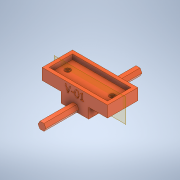
# Autodesk Inventor part: connectorToTubeBracketWithOffsetHexShaft-V01
Saved by Autodesk Inventor 2021.2 (Build 252289000, 289)
## iProperties
Created: 2020-07-23
Part Number: connectorToTubeBracketWithOffsetHexShaft-V01
Material: PBT Plastic
Document SubType Name: Modeling
Designer: robst
Density: 1.31 g/cm^3
Appearance: Smooth - Light Orange
Mass: 251.144 g
Surface Area: 396.963 cm^2
Volume: 251.144 cm^3
Author: robst
Autodesk Inventor part; units mm, degrees
ref_plane "YZ Plane" through (0, 0, 0) normal (1, 0, 0) x (0, 1, 0)
ref_plane "XZ Plane" through (0, 0, 0) normal (0, 1, 0) x (-1, 0, 0)
sketch "Sketch1" plane through (0, 0, 0) normal (0, 1, 0) x (-1, 0, 0)
  line L0 (53.975, 21.59) -> (-53.975, 21.59)
  line L1 (-53.975, 21.59) -> (-53.975, -21.59)
  line L2 (-53.975, -21.59) -> (53.975, -21.59)
  line L3 (53.975, -21.59) -> (53.975, 21.59)
  line L4 (53.975, 21.59) -> (-53.975, -21.59) construction
  line L5 (-53.975, 21.59) -> (53.975, -21.59) construction
  line L6 (60.325, 27.94) -> (-60.325, 27.94)
  line L7 (-60.325, 27.94) -> (-60.325, -27.94)
  line L8 (-60.325, -27.94) -> (60.325, -27.94)
  line L9 (60.325, -27.94) -> (60.325, 27.94)
  line L10 (60.325, 27.94) -> (-60.325, -27.94) construction
  line L11 (-60.325, 27.94) -> (60.325, -27.94) construction
  point P0 (0, 0)
  dimension "d0" = 43.18
  dimension "d1" = 107.95
  dimension "d2" = 6.35
  dimension "d3" = 6.35
  constraints: 24 end point, 4 midpoint, 4 parallel, 2 horizontal, 2 perpendicular
  measures "d0" distance of L0.end L1.end
  measures "d1" distance between parallel lines of L1 L3
  measures "d2" distance between parallel lines of L8 L2
  measures "d3" distance between parallel lines of L9 L3
extrude "Extrusion1" add sketch "Sketch1" against normal blind 12.065 contours L3 L2 L1 L0 | L9 L8 L7 L6
extrude "Extrusion2" add sketch "Sketch1" along normal blind 8.89
sketch "Sketch2" plane through (0, 0, 0) normal (0, 1, 0) x (1, 0, 0)
  line L0 (-53.975, 21.59) -> (-53.975, -21.59) construction
  line L1 (-53.975, 0) -> (53.975, 0) construction
  line L2 (53.975, -21.59) -> (53.975, 21.59) construction
  point P0 (0, 0)
  point P1 (-41.275, 0)
  point P2 (41.275, 0)
  dimension "d8" = 12.7
  dimension "d9" = 12.7
  constraints: 2 end point, 2 midpoint, 2 point on line
  measures "d8" distance from line of point (-41.275, 0) L0
  measures "d9" distance from line of point (41.275, 0) L2
hole "Hole1" at (-41.275, 0, 0) at (41.275, 0, 0) direction (0, -1, 0) diameter 5.1054 end through all counterbore diameter 10.16 counterbore depth 2.54 clearance for "Hex Machine Screw" size "#10" standard "Ansi Unified Screw Threads"
sketch "Sketch5" plane through (0, -12.065, 0) normal (0, -1, 0) x (1, 0, 0)
  line L0 (-25.4, -27.94) -> (25.4, -27.94)
  line L1 (25.4, -27.94) -> (25.4, 27.94)
  line L2 (25.4, 27.94) -> (-25.4, 27.94)
  line L3 (-25.4, 27.94) -> (-25.4, -27.94)
  line L4 (-25.4, -27.94) -> (25.4, 27.94) construction
  line L5 (25.4, -27.94) -> (-25.4, 27.94) construction
  point P0 (0, 0)
  dimension "d27" = 50.8
  dimension "d28" = 55.88
  constraints: 12 end point, 2 midpoint, 2 parallel, 1 horizontal, 1 perpendicular
  measures "d27" distance between parallel lines of L1 L3
  measures "d28" distance between parallel lines of L0 L2
extrude "Extrusion6" add sketch "Sketch5" along normal blind 19.05
sketch "Sketch11" plane through (-60.325, 8.89, 27.94) normal (0, 0, 1) x (1, 0, 0)
  line L0 (0, -20.955) -> (0, 0) construction
  line L1 (0, -10.4775) -> (120.65, -10.4775) construction
  line L2 (120.65, 0) -> (120.65, -20.955) construction
  line L3 (52.9098, -4.1275) -> (48.5358, -16.8275)
  line L4 (48.5358, -16.8275) -> (46.7142, -16.8275)
  line L5 (46.7142, -16.8275) -> (42.3402, -4.1275)
  line L6 (42.3402, -4.1275) -> (44.1515, -4.1275)
  line L7 (44.1515, -4.1275) -> (47.6713, -14.6765)
  line L8 (47.6713, -14.6765) -> (51.1911, -4.1275)
  line L9 (51.1911, -4.1275) -> (52.9098, -4.1275)
  line L10 (58.56, -12.0418) -> (53.7537, -12.0418)
  line L11 (53.7537, -12.0418) -> (53.7537, -10.4981)
  line L12 (53.7537, -10.4981) -> (58.56, -10.4981)
  line L13 (58.56, -10.4981) -> (58.56, -12.0418)
  spline S0 degree 2 poles (68.1519, -10.4775) (68.1519, -13.8944) (66.1656, -17.0951) (64.0969, -17.0951) knots 0 0 0 1 2 2 2
  spline S1 degree 2 poles (64.0969, -17.0951) (61.9974, -17.0951) (60.0317, -13.8326) (60.0317, -10.4878) knots 0 0 0 1 2 2 2
  spline S2 degree 2 poles (60.0317, -10.4878) (60.0317, -7.0504) (62.018, -3.8702) (64.0969, -3.8702) knots 0 0 0 1 2 2 2
  spline S3 degree 2 poles (64.0969, -3.8702) (66.1861, -3.8702) (68.1519, -7.1636) (68.1519, -10.4775) knots 0 0 0 1 2 2 2
  spline S4 degree 2 poles (65.97, -14.3472) (66.217, -13.7194) (66.4229, -11.7846) (66.4229, -10.4775) knots 0 0 0 1 2 2 2
  spline S5 degree 2 poles (66.4229, -10.4775) (66.4229, -9.1704) (66.217, -7.2459) (65.9597, -6.5975) knots 0 0 0 1 2 2 2
  spline S6 degree 2 poles (65.9597, -6.5975) (65.7024, -5.9491) (64.8071, -5.2802) (64.0969, -5.2802) knots 0 0 0 1 2 2 2
  spline S7 degree 2 poles (64.0969, -5.2802) (63.3868, -5.2802) (62.4708, -5.9491) (62.2032, -6.6181) knots 0 0 0 1 2 2 2
  spline S8 degree 2 poles (62.2032, -6.6181) (61.9459, -7.2665) (61.7607, -9.2425) (61.7607, -10.4878) knots 0 0 0 1 2 2 2
  spline S9 degree 2 poles (61.7607, -10.4878) (61.7607, -11.8257) (61.9254, -13.6165) (62.193, -14.3163) knots 0 0 0 1 2 2 2
  spline S10 degree 2 poles (62.193, -14.3163) (62.44, -14.975) (63.3559, -15.6851) (64.0969, -15.6851) knots 0 0 0 1 2 2 2
  spline S11 degree 2 poles (64.0969, -15.6851) (64.7968, -15.6851) (65.7127, -15.0162) (65.97, -14.3472) knots 0 0 0 1 2 2 2
  line L14 (76.9719, -16.8275) -> (70.7763, -16.8275)
  line L15 (70.7763, -16.8275) -> (70.7763, -15.5307)
  line L16 (70.7763, -15.5307) -> (73.0816, -15.5307)
  line L17 (73.0816, -15.5307) -> (73.0816, -7.0195)
  line L18 (73.0816, -7.0195) -> (70.7763, -7.0195)
  line L19 (70.7763, -7.0195) -> (70.7763, -5.8565)
  spline S12 degree 2 poles (70.7763, -5.8565) (72.0833, -5.8565) (73.3183, -5.1155) (73.4006, -4.0863) knots 0 0 0 1 2 2 2
  line L20 (73.4006, -4.0863) -> (74.718, -4.0863)
  line L21 (74.718, -4.0863) -> (74.718, -15.5307)
  line L22 (74.718, -15.5307) -> (76.9719, -15.5307)
  line L23 (76.9719, -15.5307) -> (76.9719, -16.8275)
  point P0 (60.325, -8.89)
  constraints: 2 end point, 2 midpoint, 1 horizontal
extrude "Extrusion8" cut sketch "Sketch11" against normal blind 2.54
sketch "Sketch12" plane through (-60.325, 8.89, 27.94) normal (0, 0, 1) x (1, 0, 0)
  line L0 (85.725, -40.005) -> (34.925, -40.005) construction
  line L1 (60.325, -40.005) -> (60.325, -0.5585) construction
  line L2 (63.9912, -40.005) -> (56.6588, -40.005)
  line L3 (56.6588, -40.005) -> (52.9927, -33.655)
  line L4 (52.9927, -33.655) -> (56.6588, -27.305)
  line L5 (56.6588, -27.305) -> (63.9912, -27.305)
  line L6 (63.9912, -27.305) -> (67.6573, -33.655)
  line L7 (67.6573, -33.655) -> (63.9912, -40.005)
  point P0 (60.325, -8.89)
  point P1 (60.325, -33.655)
  dimension "d86" = 12.7
  constraints: 14 end point, 1 collinear, 1 midpoint, 1 point on line, 1 vertical, 13 other
  measures "d86" distance between parallel lines of L0 L5
extrude "Extrusion9" add sketch "Sketch12" along normal blind 60.96
mirror "Mirror5" about plane through (0, 0, 0) normal (0, 0, 1) of "Extrusion9"
equation "\"d0\" = innerWidth"
equation "\"d1\" = innerLength"
equation "\"d2\" = wallThickness"
equation "\"d3\" = wallThickness"
equation "\"d4\" = bottomThickness"
equation "\"d6\" = innerDepth"
equation "\"d8\" = holeCenterFromInnerWall"
equation "\"d9\" = holeCenterFromInnerWall"
equation "\"d27\" = lowerPostLength"
equation "\"d28\" = lowerPostWidth"
equation "\"d29\" = lowerPostHeight"
equation "\"d86\" = hexSize"
equation "\"innerWidth\" = 43.18"
equation "\"innerLength\" = 107.95"
equation "\"innerDepth\" = 8.89"
equation "\"wallThickness\" = 6.35"
equation "\"postDiameter\" = 9.525"
equation "\"holeCenterFromInnerWall\" = 12.7"
equation "\"bottomThickness\" = 12.065"
equation "\"d17\" = postDiameter"
equation "\"exteriorWidth\" = innerWidth + 2 * wallThickness"
equation "\"exteriorLength\" = innerLength + 2 * wallThickness"
equation "\"exteriorHeight\" = innerDepth + bottomThickness"
equation "\"d24\" = postDiameter"
equation "\"lowerPostWidth\" = exteriorWidth"
equation "\"lowerPostLength\" = 50.8"
equation "\"lowerPostCenterX\" = 0.5 * exteriorLength"
equation "\"lowerPostHeight\" = 19.05"
equation "\"lowerPostCenterY\" = postDiameter"
equation "\"setScrewCenters\" = 0.333333 * exteriorWidth"
equation "\"hexSize\" = 12.7"
body "Solid1"
